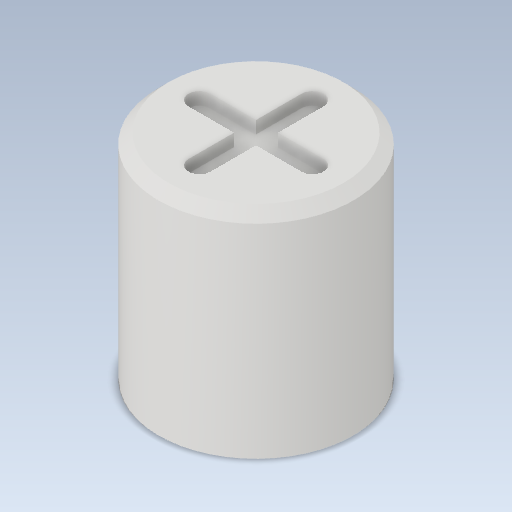
# Autodesk Inventor part: Filtr HOT 3P -korek
Saved by Autodesk Inventor 2020 (Build 240168000, 168)
## iProperties
Created: 2019-03-28
Part Number: Filtr HOT 3P -korek
Material: Tworzywo sztuczne PBT
Document SubType Name: Modeling
Designer: Marcin Kret
Mass: 2.97051 g
Surface Area: 15.8827 cm^2
Volume: 2.26756 cm^3
Density: 1.31 g/cm^3
Appearance: Gładki - biały
Author: Marcin Kret
Autodesk Inventor part; units mm, degrees
ref_plane "YZ Plane" through (0, 0, 0) normal (1, 0, 0) x (0, 1, 0)
ref_plane "XZ Plane" through (0, 0, 0) normal (0, 1, 0) x (-1, 0, 0)
ref_plane "XY Plane" through (0, 0, 0) normal (0, 0, 1) x (1, 0, 0)
sketch "Szkic1" plane through (0, 0, 0) normal (0, 1, 0) x (-1, 0, 0)
  circle A0 centre (0, 0) radius 7.75
  dimension "d0" = 15.5
  constraints: 1 centre point, 1 coincident
  measures "d0" diameter of A0
extrude "Wyciągnięcie proste1" add sketch "Szkic1" along normal blind 17
hole "Otwór1" at (0, 0, 0) direction (0, 1, 0) diameter 9.728 depth 12 thread size "7/16-20 UNF" class "2B" standard "ANSI Unified Screw Threads"
chamfer "Faza1" distance 0.8 angle 45 1 edges at (7.75, 17, 0)
sketch "Szkic2" plane through (0, 17, 0) normal (0, 1, 0) x (1, 0, 0)
  circle A0 centre (0, 0) radius 6.95 projected
  line L0 (-4.5, 0) -> (4.5, 0) construction
  line L1 (-4.5, -0.875) -> (4.5, -0.875)
  line L2 (4.5, 0.875) -> (-4.5, 0.875)
  arc A1 (-4.5, 0.875) -> (-4.5, -0.875) centre (-4.5, 0) ccw
  arc A2 (4.5, -0.875) -> (4.5, 0.875) centre (4.5, 0) ccw
  point P0 (0, 0.875)
  dimension "d15" = 1.75
  dimension "d16" = 9
  constraints: 8 end point, 4 point on circle, 4 tangent, 2 centre point, 2 midpoint, 1 coincident, 1 horizontal, 1 parallel, 1 vertical alignment
  measures "d15" diameter of A2
  measures "d16" distance of L2.start L2.end
extrude "Wyciągnięcie proste2" cut sketch "Szkic2" against normal blind 1 contours A1 L2 A2 L1
pattern_circular "Szyk kołowy1" count 4 over 360 about axis through (0, 0, 0) along (0, 1, 0) of "Wyciągnięcie proste2"
